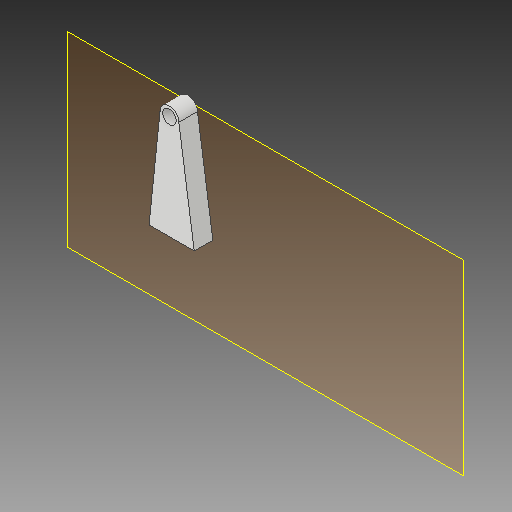
# Autodesk Inventor part: ARM
Saved by Autodesk Inventor 2017 (Build 210142000, 142)
## iProperties
Created: 2017-12-26
Part Number: ARM
Material: Generic
Document SubType Name: Modeling
Designer: will
Density: 1 g/cm^3
Appearance: Default
Author: will
Autodesk Inventor part; units mm, degrees
ref_plane "YZ Plane" through (0, 0, 0) normal (1, 0, 0) x (0, 1, 0)
ref_plane "XZ Plane" through (0, 0, 0) normal (0, 1, 0) x (-1, 0, 0)
ref_plane "XY Plane" through (0, 0, 0) normal (0, 0, 1) x (1, 0, 0)
ref_plane "Work Plane1" through (0, 0, 0) normal (0, 0, 1) x (1, 0, 0)
sketch "Sketch1" plane through (0, 0, 0) normal (0, 0, 1) x (1, 0, 0)
  ellipse E0 centre (16.5596, -41.4917) end of major axis (15.7549, -41.4917) minor radius 0.8047 projected
  circle A0 centre (16.5596, -41.4917) radius 1.086
  arc A1 (18.0749, -41.4917) -> (15.0443, -41.4917) centre (16.5596, -41.4917) ccw
  line L0 (15.0443, -41.4917) -> (13.2815, -58.1931)
  line L1 (13.2815, -58.1931) -> (20.558, -58.1931)
  line L2 (20.558, -58.1931) -> (18.0749, -41.4917)
  point P0 (0, 0)
  constraints: 6 end point, 2 centre point, 2 coincident, 2 point on circle, 1 horizontal, 1 other
extrude "Extrusion1" add sketch "Sketch1" along normal blind 3 contours L2 L1 L0 A1
body "Solid1"
